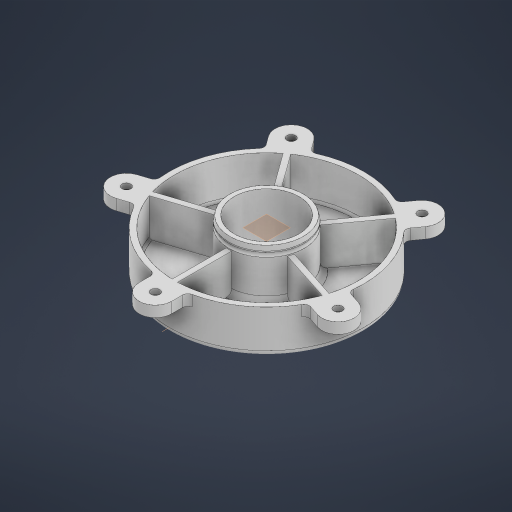
# Autodesk Inventor part: Część26
Saved by Autodesk Inventor 2023 (Build 270158000, 158)
## iProperties
Created: 2023-05-09
Part Number: Część26
Material: Ogólny
Document SubType Name: Modeling
Designer: Adam
Density: 1 g/cm^3
Appearance: Domyślna
Author: Adam
Autodesk Inventor part; units mm, degrees
ref_plane "YZ Plane" through (0, 0, 0) normal (1, 0, 0) x (0, 1, 0)
ref_plane "XZ Plane" through (0, 0, 0) normal (0, 1, 0) x (-1, 0, 0)
ref_plane "XY Plane" through (0, 0, 0) normal (0, 0, 1) x (1, 0, 0)
sketch "Szkic1" plane through (0, 0, 0) normal (0, 1, 0) x (-1, 0, 0)
  circle A0 centre (0, 0) radius 90
  circle A1 centre (0, 0) radius 30
  dimension "d0" = 180
  dimension "d1" = 60
  constraints: 2 centre point, 2 coincident
  measures "d0" diameter of A0
  measures "d1" diameter of A1
extrude "Wyciągnięcie proste1" add sketch "Szkic1" along normal blind 5
sketch "Szkic2" plane through (0, 0, 0) normal (1, 0, 0) x (0, 1, 0)
  line L0 (5, 30) -> (5, -30) projected
  line L1 (5, 30) -> (50, 30)
  line L2 (50, 30) -> (50, 34)
  line L3 (46, 35) -> (5, 35)
  line L4 (5, 35) -> (5, 30)
  line L5 (50, 34) -> (46, 35)
  circle A0 centre (43, 36.49) radius 2.49
  line L6 (60, 0) -> (-10, 0) projected
  point P0 (0, 0)
  point P1 (50, 35)
  point P2 (50, 32)
  point P3 (44.995, 35)
  point P4 (41.005, 35)
  dimension "d4" = 45
  dimension "d5" = 1
  dimension "d6" = 4
  dimension "d7" = 4.98
  dimension "d8" = 7
  dimension "d9" = 1.49
  constraints: 10 end point, 2 parallel, 2 point on line, 1 centre point, 1 horizontal, 1 midpoint, 1 perpendicular
  measures "d4" distance of L3.end point (50, 35)
  measures "d5" distance of L2.end point (50, 35)
  measures "d6" distance of L3.start point (50, 35)
  measures "d7" diameter of A0
  measures "d8" horizontal distance of A0.centre point (50, 32)
  measures "d9" distance from line of L3 A0.centre
revolve "Obrót1" add sketch "Szkic2" angle 360 about axis through (0, 5, 0) along (0, -1, 0) contours L4 L3 A0 L5 L2 L1
sketch "Szkic3" plane through (0, 0, 0) normal (1, 0, 0) x (0, 1, 0)
  line L0 (5, -90) -> (5, 90) projected
  line L1 (5, 90) -> (40, 90)
  line L2 (40, 90) -> (40, 85)
  line L3 (40, 85) -> (5, 85)
  line L4 (5, 85) -> (5, 90)
  line L5 (48, 0) -> (-8, 0) projected
  line L6 (0, -90) -> (0, 90) projected
  point P0 (0, 0)
  point P1 (40, 87.5)
  dimension "d12" = 5
  dimension "d31" = 40
  constraints: 8 end point, 2 parallel, 1 horizontal, 1 midpoint, 1 perpendicular
  measures "d12" distance of L1.end L2.end
  measures "d31" distance from line of L6 point (40, 87.5)
revolve "Obrót2" add sketch "Szkic3" angle 360 about axis through (0, 5, 0) along (0, -1, 0)
fillet "Zaokrąglenie1" radius 5 1 edges at (90, 0, 0)
fillet "Zaokrąglenie2" radius 2 1 edges at (0, 5, -85)
fillet "Zaokrąglenie3" radius 5 1 edges at (0, 5, -35)
ref_plane "Płaszczyzna konstrukcyjna3" through (0, 40, 0) normal (0, 1, 0) x (1, 0, 0)
sketch "Szkic8" plane through (0, 40, 0) normal (0, 1, 0) x (1, 0, 0)
  circle A0 centre (0, -103) radius 15
  line L0 (-15, -103) -> (-15, -83.666)
  circle A1 centre (0, 0) radius 85 projected
  line L1 (15, -103) -> (15, -83.666)
  arc A2 (-15, -83.666) -> (15, -83.666) centre (0, 0) ccw
  dimension "d40" = 30
  dimension "d41" = 103
  constraints: 6 point on circle, 4 end point, 2 centre point, 1 concentric, 1 parallel, 1 tangent, 1 vertical
  measures "d40" diameter of A0
  measures "d41" distance of A0.centre point (0, 0)
extrude "Wyciągnięcie proste3" add sketch "Szkic8" against normal blind 10 contours A0 | A0 L0 A1 L1
fillet "Zaokrąglenie5" radius 5 2 edges at (-15, 35, 88.7412) (15, 35, 88.7412)
sketch "Szkic9" plane through (0, 30, 0) normal (0, -1, 0) x (1, 0, 0)
  arc A0 (15, 103) -> (-15, 103) centre (0, 103) ccw projected
  point P0 (0, 0)
  constraints: 1 coincident
hole "Otwór2" at (0, 30, 103) direction (0, 1, 0) diameter 8 end through all counterbore diameter 15 counterbore depth 5
sketch "Szkic10" plane through (0, 40, 103) normal (0, 1, 0) x (1, 0, 0)
  circle A0 centre (0, 103) radius 85 projected
  line L0 (0, 18) -> (0, 68)
  circle A1 centre (0, 103) radius 35 projected
  constraints: 2 end point, 2 vertical alignment, 1 vertical, 2 other
rib "Żebro2" sketch "Szkic10" thickness 5 direction (0, -1, 0) end up to next extend profile yes curves L0
pattern_circular "Szyk kołowy1" count 5 over 360 about axis through (0, 5, 0) along (0, -1, 0) of "Wyciągnięcie proste3", "Żebro2", "Zaokrąglenie5", "Otwór2"
